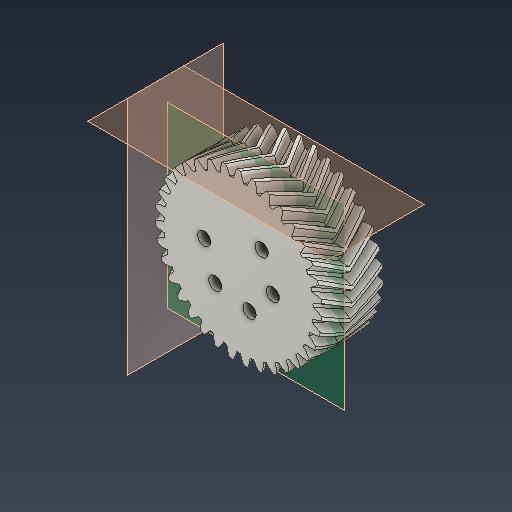
# Autodesk Inventor part: Цилиндрическое зубчатое зацепление1
Saved by Autodesk Inventor 2025 (Build 290162000, 162)
## iProperties
CustomPartVersion: 0
Created: 2025-09-24
Part Number: Цилиндрическое зубчатое зацепление1
Material: Steel
Document SubType Name: Modeling
Designer: GameHD
Categories: <?xml version="1.0" encoding="UTF-16"?> <MemberInstance><Categories><FamilyTemplate><FamilyTemplateParameter ValueType="xs:double" Id="1" ObjectReferenceKey="da_z" ObjectType="kUserParameterObject"/><FamilyTemplateParameter ValueType="xs:double" Id="2" ObjectReferenceKey="da_b" ObjectType="kUserParameterObject"/><FamilyTemplateParameter ValueType="xs:double" Id="3" ObjectReferenceKey="da_beta" ObjectType="kUserParameterObject"/><FamilyTemplateParameter ValueType="xs:double" Id="4" ObjectReferenceKey="da_da" ObjectType="kUserParameterObject"/><FamilyTemplateParameter ValueType="xs:double" Id="5" ObjectReferenceKey="da_aw" ObjectType="kUserParameterObject"/><FamilyTemplateParameter ValueType="xs:string" Id="6" ObjectReferenceKey="EAIAABAAAACIAQAAAAAAAIAAAAAAAAAA" ObjectType="83910656" SubObjectId="SurfaceGeometry"/></FamilyTemplate><ParamToTemplateMap><ParamToTemplate CategoryParameter="//CategoryParameter[@InternalName='046C89C9-8512-4d59-83FE-43B91F4F132A']" TemplateParameter="1"/><ParamToTemplate CategoryParameter="//CategoryParameter[@InternalName='2552DF32-E462-4b46-AEBF-C6C7768E72AC']" TemplateParameter="2"/><ParamToTemplate CategoryParameter="//CategoryParameter[@InternalName='C9EE641D-15FC-4fae-A226-E94C4372FDD7']" TemplateParameter="3"/><ParamToTemplate><ParamToTemplate CategoryParameter="//CategoryParameter[@InternalName='00B6519A-459B-49c7-AD84-2E56D39A5744']" ConstantValue="0.000000"/></ParamToTemplate><ParamToTemplate><ParamToTemplate CategoryParameter="//CategoryParameter[@InternalName='04B31F0E-C7A6-4894-AA32-9629BEFACF47']" ConstantValue="1.000000"/></ParamToTemplate><ParamToTemplate><ParamToTemplate CategoryParameter="//CategoryParameter[@InternalName='43CBEC2E-7847-49e7-A936-2F7889FCB2D9']" ConstantValue="0.250000"/></ParamToTemplate><ParamToTemplate><ParamToTemplate CategoryParameter="//CategoryParameter[@InternalName='B1EFC894-105D-4ebd-86BF-FA20ED196853']" ConstantValue="0.350000"/></ParamToTemplate><ParamToTemplate><ParamToTemplate CategoryParameter="//CategoryParameter[@InternalName='51175063-3D10-4879-93E8-6246FE8B403D']" ConstantValue="2060000000.000000"/></ParamToTemplate><ParamToTemplate><ParamToTemplate CategoryParameter="//CategoryParameter[@InternalName='A3A52E27-4454-46a9-B0BD-C932399B70AF']" ConstantValue="0.300000"/></ParamToTemplate><ParamToTemplate><ParamToTemplate CategoryParameter="//CategoryParameter[@InternalName='91B76062-C214-41d9-B1B9-14D2AB99603D']" ConstantValue="3.600000"/></ParamToTemplate><ParamToTemplate><ParamToTemplate CategoryParameter="//CategoryParameter[@InternalName='374E806E-8B8A-4dda-A9AA-1039D6500AD2']" ConstantValue="0.277778"/></ParamToTemplate><ParamToTemplate><ParamToTemplate CategoryParameter="//CategoryParameter[@InternalName='2D373A89-B862-43d6-8D0B-0CBF12AB9F6C']" ConstantValue="0.349066"/></ParamToTemplate><ParamToTemplate CategoryParameter="//CategoryParameter[@InternalName='37777632-D6A2-4fac-9D53-DB8ACD95C989']" TemplateParameter="4"/><ParamToTemplate CategoryParameter="//CategoryParameter[@InternalName='FD1017F1-B727-4f7e-9707-0F86F1FF9423']" TemplateParameter="5"/><ParamToTemplate><ParamToTemplate CategoryParameter="//CategoryParameter[@InternalName='9E1B4470-B2D3-4ff1-B813-535BB4CDF51A']" ConstantValue="3520000.000000"/></ParamToTemplate><ParamToTemplate><ParamToTemplate CategoryParameter="//CategoryParameter[@InternalName='F8452263-BFF6-458c-9FB1-07C4B99E95CD']" ConstantValue="11400000.000000"/></ParamToTemplate><ParamToTemplate><ParamToTemplate CategoryParameter="//CategoryParameter[@InternalName='3E3BB259-FD49-497f-8171-6EBC954A3479']" ConstantValue="2.000000"/></ParamToTemplate><ParamToTemplate CategoryParameter="//CategoryParameter[@InternalName='27C3BAF2-7550-4e4b-AE2C-0DB134B7D9B7']" TemplateParameter="6"/></ParamToTemplateMap><Category DisplayName="Gear" InternalName="DC85795E-93AB-48d5-8EEE-5A27447B64BD" Mnemonic="Gear"><CategoryParameter DisplayName="z" InternalName="046C89C9-8512-4d59-83FE-43B91F4F132A" Mnemonic="z"/><CategoryParameter DisplayName="b" InternalName="2552DF32-E462-4b46-AEBF-C6C7768E72AC" Mnemonic="b"/><CategoryParameter DisplayName="||b|" InternalName="C9EE641D-15FC-4fae-A226-E94C4372FDD7" Mnemonic="beta"/><CategoryParameter DisplayName="x" InternalName="00B6519A-459B-49c7-AD84-2E56D39A5744" Mnemonic="x"/><CategoryParameter DisplayName="a*" InternalName="04B31F0E-C7A6-4894-AA32-9629BEFACF47" Mnemonic="a"/><CategoryParameter DisplayName="c*" InternalName="43CBEC2E-7847-49e7-A936-2F7889FCB2D9" Mnemonic="c"/><CategoryParameter DisplayName="r|.f|*" InternalName="B1EFC894-105D-4ebd-86BF-FA20ED196853" Mnemonic="rf"/><CategoryParameter DisplayName="E" InternalName="51175063-3D10-4879-93E8-6246FE8B403D" Mnemonic="E"/><CategoryParameter DisplayName="||m|" InternalName="A3A52E27-4454-46a9-B0BD-C932399B70AF" Mnemonic="mi"/><Category DisplayName="SpurGear" InternalName="26C5A22E-A91E-4dfd-A3B3-23CCAFAE1764" Mnemonic="SpurGear"><CategoryParameter DisplayName="m" InternalName="91B76062-C214-41d9-B1B9-14D2AB99603D" Mnemonic="m"/><CategoryParameter DisplayName="P" InternalName="374E806E-8B8A-4dda-A9AA-1039D6500AD2" Mnemonic="PP"/><CategoryParameter DisplayName="||a|" InternalName="2D373A89-B862-43d6-8D0B-0CBF12AB9F6C" Mnemonic="alpha"/><CategoryParameter DisplayName="d|.a|" InternalName="37777632-D6A2-4fac-9D53-DB8ACD95C989" Mnemonic="da"/><CategoryParameter DisplayName="a|.w|" InternalName="FD1017F1-B727-4f7e-9707-0F86F1FF9423" Mnemonic="aw"/><CategoryParameter DisplayName="||s||.Flim|" InternalName="9E1B4470-B2D3-4ff1-B813-535BB4CDF51A" Mnemonic="sFlim"/><CategoryParameter DisplayName="||s||.Hlim|" InternalName="F8452263-BFF6-458c-9FB1-07C4B99E95CD" Mnemonic="sHlim"/><CategoryParameter DisplayName="тип" InternalName="3E3BB259-FD49-497f-8171-6EBC954A3479" Mnemonic="type"/><CategoryParameter DisplayName="PitchDiameter" InternalName="27C3BAF2-7550-4e4b-AE2C-0DB134B7D9B7" Mnemonic="IDS_PITCHDIAM"/></Category></Category></Categories></MemberInstance>
Density: 1 g/cm^3
Appearance: Steel
d16: 36,000 мм
d17: 0,000 мм
d41: 0,000 мм
d43: 36,000 мм
d46: 36,000 мм
d47: 0,000 мм
d48: 0,000 мм
Author: GameHD
Autodesk Inventor part; units mm, degrees
ref_plane "YZ Plane" through (0, 0, 0) normal (1, 0, 0) x (0, 1, 0)
ref_plane "XY Plane" through (0, 0, 0) normal (0, 0, 1) x (1, 0, 0)
sketch "Sketch1" plane through (0, 0, 0) normal (0, 0, 1) x (1, 0, 0)
  circle A0 centre (0, 0) radius 19.0857
  dimension "d0" = 38.1713
  constraints: 1 centre point
  measures "d0" diameter of A0
extrude "Extrusion1" add sketch "Sketch1" along normal blind 7
ref_plane "Work Plane2" through (0, 0, 3.5) normal (0, 0, 1) x (1, 0, 0)
sketch "Sketch2" plane through (0, 0, 0) normal (0, 0, -1) x (-1, 0, 0)
  circle A0 centre (0, 0) radius 19.0857 projected
  circle A1 centre (0, 0) radius 18.1865
  dimension "d3" = 36.3731
  constraints: 1 centre point, 1 coincident
  measures "d3" diameter of A1
surface extrude "Средний диаметр" sketch "Sketch2" against normal through all shown no curves A1
ref_plane "Work Plane8" through (0, 0, 0) normal (0.9959743, 0.0896393, 0) x (0, 0, 1)
ref_plane "Work Plane9" through (0, 0, 0) normal (1, 0, 0) x (0, 1, 0)
spur gear teeth "Цилиндрическое зубчатое зацепление" teeth 35 pitch diameter 36.3731 tip diameter 38.1713 root diameter 34.1231 face width 7 helix angle 30 hand left start plane through (0, 0, 0) normal (0, 0, -1) x (-1, 0, 0)
mirror "Зеркальное отражение2" about plane through (0, 0, 7) normal (0, 0, 1) of "Extrusion1", "Цилиндрическое зубчатое зацепление"
ref_plane "РабПлоскость11" through (0, 0, 13) normal (0, 0, 1) x (1, 0, 0)
ref_plane "РабПлоскость12" through (0, 0, 10) normal (0, 0, -1) x (-1, 0, 0)
ref_plane "РабПлоскость13" through (-18.5, 0, 0) normal (1, 0, 0) x (0, 1, 0)
ref_plane "РабПлоскость14" through (0, 18.5, 0) normal (0, 1, 0) x (-1, 0, 0)
sketch "Эскиз14" plane through (0, 0, 14) normal (0, 0, 1) x (0.9485364, 0.316668, 0)
  circle A0 centre (6.9282, -4) radius 1.5
  circle A1 centre (0, -8) radius 1.5
  circle A2 centre (6.9282, 4) radius 1.5
  circle A3 centre (-6.9282, -4) radius 1.5
  circle A4 centre (-6.9282, 4) radius 1.5
  circle A5 centre (0, -8) radius 1.5
  circle A6 centre (6.9282, -4) radius 1.5
  circle A7 centre (6.9282, 4) radius 1.5
  circle A8 centre (-6.9282, 4) radius 1.5
  circle A9 centre (-6.9282, -4) radius 1.5
  point P0 (0, 0)
  point P1 (0, 0)
  point P2 (0, 0)
  point P3 (-0.0002, -0.0007)
  point P4 (0, 0)
  point P5 (-0.0001, -0.0007)
  point P6 (0, 0)
  point P7 (0, -0.0007)
  point P8 (0, 0)
  point P9 (0.0002, -0.0007)
  point P10 (0, 0)
  point P11 (0.0003, -0.0007)
  point P12 (0, 0)
  point P13 (0.0004, -0.0006)
  point P14 (0, 0)
  point P15 (0.0005, -0.0005)
  point P16 (0, 0)
  point P17 (0.0005, -0.0005)
  point P18 (0, 0)
  point P19 (0.0006, -0.0004)
  point P20 (0, 0)
  point P21 (0.0007, -0.0003)
  point P22 (0, 0)
  point P23 (0.0007, -0.0002)
  point P24 (0, 0)
  point P25 (0.0007, 0)
  point P26 (0, 0)
  point P27 (0.0007, 0.0001)
  point P28 (0, 0)
  point P29 (0.0007, 0.0002)
  point P30 (0, 0)
  point P31 (0.0007, 0.0003)
  point P32 (0, 0)
  point P33 (0.0006, 0.0004)
  point P34 (0, 0)
  point P35 (0.0005, 0.0005)
  point P36 (0, 0)
  point P37 (0.0004, 0.0006)
  point P38 (0, 0)
  point P39 (0.0003, 0.0006)
  point P40 (0, 0)
  point P41 (0.0002, 0.0007)
  point P42 (0, 0)
  point P43 (0.0001, 0.0007)
  point P44 (0, 0)
  point P45 (0, 0.0007)
  point P46 (0, 0)
  point P47 (-0.0001, 0.0007)
  point P48 (0, 0)
  point P49 (-0.0002, 0.0007)
  point P50 (0, 0)
  point P51 (-0.0003, 0.0006)
  point P52 (0, 0)
  point P53 (-0.0004, 0.0006)
  point P54 (0, 0)
  point P55 (-0.0005, 0.0005)
  point P56 (0, 0)
  point P57 (-0.0006, 0.0004)
  point P58 (0, 0)
  point P59 (-0.0006, 0.0003)
  point P60 (0, 0)
  point P61 (-0.0007, 0.0002)
  point P62 (0, 0)
  point P63 (-0.0007, 0.0001)
  point P64 (0, 0)
  point P65 (-0.0007, 0)
  point P66 (0, 0)
  point P67 (-0.0007, -0.0001)
  point P68 (0, 0)
  point P69 (-0.0007, -0.0002)
  point P70 (0, 0)
  point P71 (-0.0006, -0.0003)
  point P72 (0, 0)
  point P73 (-0.0006, -0.0004)
  point P74 (0, 0)
  point P75 (-0.0005, -0.0005)
  point P76 (0, 0)
  point P77 (-0.0004, -0.0006)
  point P78 (0, 0)
  point P79 (-0.0003, -0.0007)
  point P80 (-0.0003, -0.0007)
  point P81 (0, 0)
  constraints: 10 centre point, 2 coincident
extrude "Выдавливание12" cut sketch "Эскиз14" against normal through all
equation "\"d0\" = da_da"
equation "\"d1\" = da_b"
equation "\"d3\" = da_d"
equation "\"d16\" = da_aw"
equation "\"d43\" = da_aw"
equation "\"d46\" = da_aw"
equation "\"da_da\" = 38.171314"
equation "\"da_b\" = 7"
equation "\"da_d\" = 36.373067"
equation "\"da_aw\" = 36"
body "Solid1"
body "Srf1"
